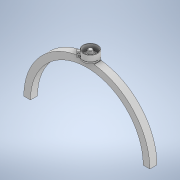
# Autodesk Inventor part: bottom_gimbal_ring
Saved by Autodesk Inventor 2022 (Build 260153000, 153)
## iProperties
Created: 2022-03-15
Part Number: bottom_gimbal_ring
Material: Generic
Document SubType Name: Modeling
Designer: kylem
Density: 1 g/cm^3
Appearance: Default
Author: kylem
Autodesk Inventor part; units mm, degrees
ref_plane "YZ Plane" through (0, 0, 0) normal (1, 0, 0) x (0, 1, 0)
ref_plane "XZ Plane" through (0, 0, 0) normal (0, 1, 0) x (-1, 0, 0)
ref_plane "XY Plane" through (0, 0, 0) normal (0, 0, 1) x (1, 0, 0)
sketch "Sketch1" plane through (0, 0, 0) normal (0, 1, 0) x (-1, 0, 0)
  circle A0 centre (0, 0) radius 16.375
  dimension "d0" = 32.75
  constraints: 1 centre point, 1 coincident
  measures "d0" diameter of A0
extrude "Extrusion1" add sketch "Sketch1" along normal blind 3
sketch "Sketch2" plane through (0, 3, 0) normal (0, 1, 0) x (1, 0, 0)
  circle A0 centre (0, 0) radius 4.75
  dimension "d3" = 9.5
  constraints: 1 centre point, 1 coincident
  measures "d3" diameter of A0
extrude "Extrusion2" add sketch "Sketch2" along normal blind 14
chamfer "Chamfer1" distance 1 angle 45 1 edges at (-4.75, 17, 0)
sketch "Sketch3" plane through (0, 3, 0) normal (0, 1, 0) x (1, 0, 0)
  circle A0 centre (0, 0) radius 15.5
  circle A1 centre (0, 0) radius 16.375
  line L0 (0, 0) -> (0, 16.375)
  circle A2 centre (0, 0) radius 16.375 projected
  line L1 (0, 0) -> (16.375, 0)
  point P0 (15.5, 0)
  point P1 (0, 15.5)
  dimension "d9" = 31
  dimension "d26" = 32.75
  constraints: 4 end point, 2 centre point, 2 coincident, 2 point on circle, 1 horizontal
  measures "d9" diameter of A0
  measures "d26" diameter of A1
extrude "Extrusion3" add sketch "Sketch3" along normal blind 13.5 contours A0 L0 A1 L1 picked at (14.8943, 5.8246)
sketch "Sketch4" plane through (0, 16.5, 0) normal (0, 1, 0) x (1, 0, 0)
  arc A0 (-10.8502, -12.2644) -> (-12.2644, -10.8502) centre (0, 0) ccw
  circle A1 centre (0, 0) radius 3.75 projected
  line L0 (0, 16.375) -> (0, 15.5) projected
  arc A2 (-10.2302, -11.6444) -> (-11.6444, -10.2302) centre (0, 0) ccw
  line L1 (0, 0) -> (-0.7071, 0.7071)
  line L2 (0, 0) -> (1, 0) construction
  line L3 (-0.7071, 0.7071) -> (0.7071, -0.7071)
  line L4 (1.0882, -0.326) -> (-18.1603, -19.5746)
  line L5 (-0.7071, 0.7071) -> (-13.3956, -11.9813)
  line L6 (-13.3956, -11.9813) -> (-11.0324, -14.3445)
  line L7 (-10.2302, -11.6444) -> (-7.7553, -14.1193)
  line L8 (-10.2302, -11.6444) -> (-6.7302, -11.6444) construction
  line L9 (-7.9511, -14.3151) -> (-11.998, -18.3619)
  line L10 (-14.4448, -7.7128) -> (-18.1483, -4.0093)
  line L11 (-11.6444, -10.2302) -> (-4.6444, -10.2302) construction
  line L12 (-18.1483, -4.0093) -> (-22.391, -8.252)
  line L13 (-18.1483, -4.0093) -> (-12.1483, -4.0093) construction
  line L14 (-13.3956, -11.9813) -> (-20.1314, -18.7172)
  line L15 (-18.1603, -19.5746) -> (-18.1603, -19.5746)
  line L16 (-18.1603, -19.5746) -> (-21.0847, -16.6502)
  line L17 (-22.391, -8.252) -> (-16.0286, -14.6144)
  line L18 (-14.4729, -15.8871) -> (-11.998, -18.3619)
  dimension "d12" = 1
  dimension "d13" = 135
  dimension "d14" = 2
  dimension "d15" = 0
  dimension "d16" = 3.5
  dimension "d17" = 45
  dimension "d18" = 6
  dimension "d19" = 90
  dimension "d20" = 9
  dimension "d21" = 135
  dimension "d22" = 6
  dimension "d23" = 135
  dimension "d29" = 16.375
  dimension "d30" = 2
  dimension "d31" = 3.5
  constraints: 36 end point, 9 perpendicular, 7 point on circle, 7 point on line, 4 horizontal, 3 equal length, 2 centre point, 2 coincident, 1 collinear
  measures "d12" distance of L1.start L1.end
  measures "d13" angle of L2 L1
  measures "d14" distance of L1.end L3.end
  measures "d15" distance between parallel lines of L3 L1
  measures "d16" distance of L7.start L7.end
  measures "d17" angle of L7 L8
  measures "d18" distance of L7.end L9.end
  measures "d19" angle of L7 L9
  measures "d20" distance of L11.start L10.end
  measures "d21" angle of L11 L10
  measures "d22" distance of L10.end L12.end
  measures "d23" angle of L12 L13
  measures "d29" radius of A0
  measures "d30" distance between parallel lines of L15 L14
  measures "d31" distance between parallel lines of L9 L4
extrude "Extrusion5" add sketch "Sketch4" against normal blind 13 contours L4 A2 L0 A0 | A0 L9 L18 L4 | L0 A2 L5 A0 | L14 L17 L12 L10 A0 L5
sketch "Sketch6" plane through (0, 16.5, 0) normal (0, 1, 0) x (1, 0, 0)
  line L0 (-11.6444, -10.2302) -> (-9.6444, -10.2302) construction
  line L1 (-22.391, -8.252) -> (-16.0286, -14.6144) projected
  line L2 (-16.0286, -14.6144) -> (-17.4428, -13.2001)
  line L3 (-16.0286, -14.6144) -> (-11.6444, -10.2302) projected
  line L4 (-16.0286, -14.6144) -> (-11.6444, -10.2302)
  line L5 (-16.0286, -14.6144) -> (-17.4428, -13.2001)
  line L6 (-16.0286, -14.6144) -> (-14.0286, -14.6144) construction
  line L7 (-17.4428, -13.2001) -> (-10.3717, -6.1291)
  line L8 (-10.3717, -6.1291) -> (-8.2504, -8.2504)
  line L9 (-10.3717, -6.1291) -> (-7.3717, -6.1291) construction
  line L10 (-8.2504, -8.2504) -> (-15.3215, -15.3215)
  line L11 (-16.0286, -14.6144) -> (-22.391, -8.252) projected
  line L12 (-15.3215, -15.3215) -> (-17.4428, -13.2001)
  line L13 (-8.252, -22.391) -> (-14.6144, -16.0286)
  line L14 (-13.2001, -17.4428) -> (-6.1291, -10.3717)
  line L15 (-6.1291, -10.3717) -> (-8.2504, -8.2504)
  line L16 (-15.3215, -15.3215) -> (-13.2001, -17.4428)
  point P0 (0, 0)
  dimension "d34" = 2
  dimension "d35" = 135
  dimension "d36" = 10
  dimension "d37" = 90
  dimension "d39" = 3
  dimension "d40" = 45
  dimension "d41" = 10
  dimension "d42" = 90
  constraints: 28 end point, 4 symmetric about line, 3 horizontal, 2 collinear, 2 equal length, 2 perpendicular, 2 point on line
  measures "d34" distance of L1.end L2.end
  measures "d35" angle of L6 L5
  measures "d36" distance of L2.end L7.end
  measures "d37" angle of L5 L7
  measures "d39" distance of L7.end L8.end
  measures "d40" angle of L8 L9
  measures "d41" distance of L8.end L10.end
  measures "d42" angle of L8 L10
extrude "Extrusion6" cut sketch "Sketch6" against normal blind 13
sketch "Sketch7" plane through (0, 16.5, 0) normal (0, 1, 0) x (1, 0, 0)
  circle A0 centre (0, 0) radius 3.75 projected
  circle A1 centre (0, 0) radius 16.375
  line L0 (-22.391, -8.252) -> (-12.1273, 2.0117)
  line L1 (-22.391, -8.252) -> (-7.876, -8.252) construction
  line L2 (-18.1483, -4.0093) -> (-14.4448, -7.7128) projected
  line L3 (-18.1483, -4.0093) -> (-14.4448, -7.7128)
  line L4 (-7.9511, -14.3151) -> (-11.998, -18.3619) projected
  line L5 (-11.998, -18.3619) -> (-9.8767, -16.2406)
  line L6 (-9.8767, -16.2406) -> (-5.4147, -15.4539)
  circle A2 centre (0, 0) radius 16.375 projected
  line L7 (-9.8767, -16.2406) -> (-7.9511, -14.3151)
  point P0 (-16.2397, -2.1007)
  dimension "d45" = 45
  dimension "d46" = 3
  dimension "d47" = 145
  constraints: 12 end point, 2 collinear, 1 centre point, 1 coincident, 1 equal length, 1 horizontal, 1 point on circle, 1 point on line
  measures "d45" angle of L1 L0
  measures "d46" distance of L4.end L5.end
  measures "d47" angle of L5 L6
extrude "Extrusion7" add sketch "Sketch7" against normal blind 13 contours L2 L0 A1 | A1 L6 L4
sketch "Sketch8" plane through (0, 16.5, 0) normal (0, 1, 0) x (1, 0, 0)
  circle A0 centre (0, 0) radius 3.75 projected
  line L0 (-13.0586, -17.3013) -> (-8.6316, -12.8742) projected
  circle A1 centre (0, 0) radius 15.5
  circle A2 centre (0, 0) radius 16.375
  arc A3 (-8.6316, -12.8742) -> (-12.8742, -8.6316) centre (0, 0) ccw projected
  circle A4 centre (0, 0) radius 27.7287
  constraints: 3 centre point, 3 coincident, 1 point on circle
extrude "Extrusion8" cut sketch "Sketch8" against normal blind 7 contours A4
chamfer "Chamfer2" distance 6 angle 45 1 edges at (-4.75, 3, 0)
sketch "Sketch9" plane through (-11.998, 3.5, 18.3619) normal (0.7071068, 0, 0.7071068) x (0.7071068, 0, -0.7071068)
  line L0 (-0.2001, 6) -> (8.4991, 6) projected
  line L1 (-0.2001, 6) -> (2.7999, 6)
  line L2 (2.7999, 6) -> (2.7999, 3)
  line L3 (3, 0) -> (3, 6) projected
  circle A0 centre (2.7999, 3) radius 1.35
  point P0 (21.4677, -3.5)
  dimension "d55" = 3
  dimension "d56" = 3
  dimension "d57" = 90
  dimension "d58" = 2.7
  constraints: 4 end point, 1 centre point, 1 coincident, 1 parallel, 1 point on line
  measures "d55" distance of L0.start L1.end
  measures "d56" distance of L1.end L2.end
  measures "d57" angle of L1 L2
  measures "d58" diameter of A0
extrude "Extrusion9" cut sketch "Sketch9" along normal mid plane 50 contours A0 L3 | A0 L3
sketch "Sketch10" plane through (-8.6316, 3.5, 12.8742) normal (-0.7071068, 0, -0.7071068) x (-0.7071068, 0, 0.7071068)
  circle A0 centre (3.4609, 3) radius 1.35 projected
  circle A1 centre (3.4609, 3) radius 1.6
  point P0 (-15.2069, -3.5)
  dimension "d61" = 3.2
  constraints: 1 centre point, 1 coincident
  measures "d61" diameter of A1
extrude "Extrusion10" cut sketch "Sketch10" against normal blind 50 contours A0 | A1
sketch "Sketch11" plane through (-11.998, 3.5, 18.3619) normal (0.7071068, 0, 0.7071068) x (0.7071068, 0, -0.7071068)
  arc A0 (3, 1.4126) -> (3, 4.5874) centre (2.7999, 3) ccw projected
  circle A1 centre (2.7999, 3) radius 3
  line L0 (3, 0) -> (0, 0) projected
  point P0 (21.4677, -3.5)
  constraints: 1 centre point, 1 coincident, 1 tangent
extrude "Extrusion11" cut sketch "Sketch11" along normal blind 50
sketch "Sketch12" plane through (0, 16.5, 0) normal (0, 1, 0) x (1, 0, 0)
  circle A0 centre (0, 0) radius 3.75 projected
  arc A1 (-9.2616, -13.5042) -> (-13.5042, -9.2616) centre (0, 0) ccw
  arc A2 (-9.5312, -13.7738) -> (-13.7738, -9.5312) centre (0, 0) ccw
  arc A3 (-8.6316, -12.8742) -> (-12.8742, -8.6316) centre (0, 0) ccw projected
  line L0 (-17.4428, -13.2001) -> (-22.391, -8.252) projected
  line L1 (-12.8742, -8.6316) -> (-17.4428, -13.2001)
  line L2 (-13.0586, -17.3013) -> (-8.6316, -12.8742) projected
  line L3 (-8.6316, -12.8742) -> (-13.0586, -17.3013)
  point P0 (-9.2616, -13.5042)
  dimension "d66" = 33.5
  constraints: 4 end point, 4 point on circle, 4 point on line, 2 centre point, 2 coincident, 1 collinear, 1 perpendicular
  measures "d66" diameter of A2
extrude "Extrusion12" add sketch "Sketch12" against normal blind 13 contours A1 L1 A2 L2
sketch "Sketch13" plane through (0, 3.5, 0) normal (0, -1, 0) x (1, 0, 0)
  circle A0 centre (0, 0) radius 16.75
  arc A1 (-13.7738, 9.5312) -> (-9.5312, 13.7738) centre (0, 0) ccw projected
  line L0 (0, -15.5) -> (0, -16.375) projected
  circle A2 centre (0, 0) radius 16.375
  line L1 (0, 0) -> (0, -16.75)
  line L2 (0, 0) -> (16.75, 0)
  point P0 (16.75, 0)
  point P1 (16.375, 0)
  constraints: 4 end point, 2 coincident, 2 point on circle, 1 centre point, 1 perpendicular, 1 vertical, 3 other
extrude "Extrusion13" add sketch "Sketch13" along normal blind 3.5 contours A0 L1 A2 L2 picked at (2.457, -16.3482)
sketch "Sketch14" plane through (0, 0, 0) normal (0, -1, 0) x (1, 0, 0)
  line L0 (0, -16.375) -> (0, -16.75) projected
  circle A0 centre (0, 0) radius 16.75
  constraints: 1 coincident, 1 vertical alignment, 2 other
extrude "Extrusion14" add sketch "Sketch14" against normal blind 3
sketch "Sketch17" plane through (0, 0, 0) normal (0, 0, 1) x (1, 0, 0)
  line L0 (0, 0) -> (0, -285)
  circle A0 centre (0, -142.5) radius 127.5
  arc A1 (-16.75, -0.9879) -> (16.75, -0.9879) centre (0, -142.5) ccw
  line L1 (0, -142.5) -> (-142.5, -142.5)
  line L2 (-142.5, -142.5) -> (142.5, -142.5)
  line L3 (-16.75, 0) -> (16.75, 0) projected
  line L4 (-16.75, 0) -> (-16.75, -2.0764)
  line L5 (16.75, 0) -> (16.75, -2.4091)
  line L6 (16.75, 0) -> (-16.75, 0)
  point P0 (-127.5, -142.5)
  point P1 (127.5, -142.5)
  dimension "d77" = 285
  dimension "d78" = 255
  dimension "d79" = 285
  constraints: 12 end point, 4 point on circle, 3 point on line, 2 centre point, 2 perpendicular, 2 vertical, 1 coincident, 1 horizontal, 1 midpoint
  measures "d77" distance of L0.start L0.end
  measures "d78" diameter of A0
  measures "d79" diameter of A1
extrude "Extrusion15" add sketch "Sketch17" along normal mid plane 16 contours L3 L5 A1 L2 A0 L0 | L0 A0 L1 A1 L4 L3
body "Solid1"
